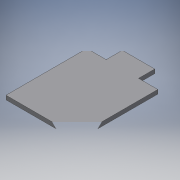
# Autodesk Inventor part: Side wall
Saved by Autodesk Inventor 2016 (Build 200138000, 138)
## iProperties
Created: 2016-04-09
Part Number: Side wall
Material: Generic
Document SubType Name: Modeling
Designer: Vijay
Density: 1 g/cm^3
Appearance: Default
Author: Vijay
Autodesk Inventor part; units mm, degrees
ref_plane "YZ Plane" through (0, 0, 0) normal (1, 0, 0) x (0, 1, 0)
ref_plane "XZ Plane" through (0, 0, 0) normal (0, 1, 0) x (-1, 0, 0)
ref_plane "XY Plane" through (0, 0, 0) normal (0, 0, 1) x (1, 0, 0)
sketch "Sketch1" plane through (0, 0, 0) normal (0, 0, 1) x (1, 0, 0)
  line L0 (-10.6243, -0.0072) -> (4.3757, -0.0072)
  line L1 (4.3757, -0.0072) -> (4.3757, -0.5072)
  line L2 (4.3757, -0.5072) -> (-10.6243, -0.5072)
  line L3 (-10.6243, -0.5072) -> (-10.6243, -0.0072)
  point P0 (0, 0)
  dimension "d0" = 0.5
  dimension "d1" = 15
  constraints: 8 end point, 2 parallel, 1 horizontal, 1 perpendicular
  measures "d0" distance of L2.end L0.start
  measures "d1" distance of L1.end L2.end
extrude "Extrusion1" add sketch "Sketch1" along normal blind 10
sketch "Sketch2" plane through (-10.6243, -0.0072, 0) normal (0, 1, 0) x (1, 0, 0)
  line L0 (0, 0) -> (15, 0) construction
  line L1 (7.5, 0) -> (7.5, -10.8529) construction
  line L2 (15, -5.4265) -> (-1.0951, -5.4265) construction
  line L3 (5.5, 2) -> (9.5, 2)
  line L4 (9.5, 2) -> (9.5, 0)
  line L5 (9.5, 0) -> (5.5, 0)
  line L6 (5.5, 0) -> (5.5, 2)
  point P0 (10.6243, 0)
  dimension "d4" = 4
  dimension "d5" = 2
  constraints: 12 end point, 2 horizontal, 2 parallel, 1 midpoint, 1 perpendicular, 1 point on line, 1 vertical, 1 other
  measures "d4" distance of L3.start L3.end
  measures "d5" distance of L5.end L3.start
extrude "Extrusion2" add sketch "Sketch2" against normal blind 0.5
sketch "Sketch3" plane through (-10.6243, -0.0072, 10) normal (0, 1, 0) x (1, 0, 0)
  line L0 (0, 10) -> (5.5, 10) projected
  line L1 (0, 10) -> (0, 0) projected
  line L2 (15, 0) -> (0, 0) projected
  line L3 (15, 10) -> (15, 0) projected
  line L4 (9.5, 10) -> (15, 10) projected
  line L5 (9.5, 12) -> (9.5, 10) projected
  line L6 (5.5, 12) -> (9.5, 12) projected
  line L7 (5.5, 10) -> (5.5, 12) projected
  line L8 (3.116, 10) -> (3.116, 0)
  line L9 (15, 0) -> (0, 0) projected
  line L10 (15, 10) -> (9.5, 10) projected
  line L11 (11.884, 10) -> (11.884, 0)
  line L12 (5.5, 12) -> (9.5, 12) construction
  line L13 (7.5, 12) -> (7.5, 0) construction
  point P0 (10.6243, 10)
  constraints: 6 end point, 4 point on line, 2 midpoint, 2 perpendicular, 1 other
extrude "Extrusion3" cut sketch "Sketch3" against normal blind 1 contours L0 L8 L2 L1 | L11 L4 L3 L2
sketch "Sketch4" plane through (-5.1243, -0.0072, -2) normal (0, 1, 0) x (1, 0, 0)
  line L0 (8.8107, -14.8925) -> (-5.1696, -14.8925)
  line L1 (-5.1696, -14.8925) -> (-5.1696, -4.6188)
  line L2 (-5.1696, -4.6188) -> (8.8107, -4.6188)
  line L3 (8.8107, -4.6188) -> (8.8107, -14.8925)
  point P0 (5.1243, -2)
  constraints: 8 end point, 2 parallel, 1 horizontal, 1 perpendicular
extrude "Extrusion4" cut sketch "Sketch4" against normal blind 1
body "Solid1"
